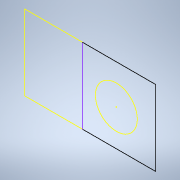
# Autodesk Inventor part: Palanca servo_dedo_2
Saved by Autodesk Inventor 2020 (Build 240168000, 168)
## iProperties
Created: 2021-08-17
Part Number: Palanca servo_dedo_2
Material: Generic
Document SubType Name: Modeling
Designer: chalo
Density: 1 g/cm^3
Appearance: Default
Author: chalo
Autodesk Inventor part; units mm, degrees
ref_plane "YZ Plane" through (0, 0, 0) normal (1, 0, 0) x (0, 1, 0)
ref_plane "XZ Plane" through (0, 0, 0) normal (0, 1, 0) x (-1, 0, 0)
ref_plane "XY Plane" through (0, 0, 0) normal (0, 0, 1) x (1, 0, 0)
sketch "Sketch1" plane through (0, 0, 0) normal (0, 0, 1) x (1, 0, 0)
  circle A0 centre (-2.5, -3) radius 1.6 projected
  line L0 (-10, -5.75) -> (0, -5.75) projected
  line L1 (0, 0) -> (0, -5.75) projected
  line L2 (-10, 0) -> (0, 0) projected
  line L3 (-10, -2) -> (-10, 0) projected
  line L4 (-10, -2) -> (-10, -3.75) projected
  line L5 (-10, -5.75) -> (-10, -3.75) projected
  line L6 (0, -5.75) -> (-5, -5.75)
  line L7 (-5, -5.75) -> (-5, 0)
  line L8 (-5, 0) -> (0, 0)
  line L9 (0, 0) -> (0, -5.75)
  dimension "d0" = 2.5
  constraints: 8 end point, 2 parallel, 1 horizontal, 1 midpoint, 1 perpendicular
  measures "d0" distance from line of A0.centre L7
extrude "Extrusion1" add sketch "Sketch1" along normal blind 4 contours L7 L2 L1 L0
sketch "Sketch2" plane through (-5, 0, 0) normal (0, 1, 0) x (1, 0, 0)
  line L0 (5, 0) -> (0, 0) projected
  line L1 (0, 0) -> (0, -4) projected
  line L2 (5, -4) -> (0, -4) projected
  line L3 (5, 0) -> (5, -4) projected
  line L4 (24.0211, -5.907) -> (18.6171, -5.907) projected
  line L5 (24.0211, -17.407) -> (18.6171, -17.407) projected
  line L6 (5, -4) -> (18.0171, -13.657)
  line L7 (5, 0) -> (18.0171, -9.657)
  line L8 (18.6171, -17.407) -> (18.6171, -13.657) construction
  line L9 (18.6171, -5.907) -> (18.6171, -9.657) construction
  line L10 (18.6171, -9.657) -> (18.6171, -13.657) construction
  line L11 (24.0211, -5.907) -> (24.0211, -17.407) construction
  line L12 (18.0171, -9.657) -> (26.5171, -9.657)
  line L13 (18.0171, -13.657) -> (26.5171, -13.657)
  line L14 (26.5171, -13.657) -> (26.5171, -9.657)
  line L15 (20.0171, -11.057) -> (20.0171, -5.657) construction
  point P0 (24.0211, -11.657)
  point P1 (18.6171, -11.657)
  dimension "d3" = 4
  dimension "d4" = 8.5
  dimension "d7" = 2
  constraints: 18 end point, 4 vertical, 3 horizontal alignment, 3 perpendicular, 2 midpoint, 1 vertical alignment
  measures "d3" distance of L9.end L8.end
  measures "d4" distance of L7.end L12.end
  measures "d7" distance from line of L15 L7.end
extrude "Extrusion2" add sketch "Sketch2" against normal blind 10 contours L7 L12 L14 L13 L6 L3
sketch "Sketch3" plane through (13.0171, 0, 13.657) normal (0, 0, 1) x (1, 0, 0)
  circle A0 centre (4.6, -6.8) radius 1.55 construction
  line L0 (-13.0171, 0) -> (0, 0) construction
  line L1 (-13.0171, -5.75) -> (-13.0171, 0) projected
  line L2 (-13.0171, -5.75) -> (-13.0171, -10) projected
  line L3 (0, -10) -> (-13.0171, -10) projected
  line L4 (0, 0) -> (0, -10) construction
  line L5 (0, 0) -> (8.5, 0) projected
  line L6 (0, 0) -> (0, -10) construction
  line L7 (8.5, -10) -> (0, -10) construction
  line L8 (8.5, 0) -> (8.5, -10) projected
  line L9 (-18.0171, -5.75) -> (-13.0171, -5.75) projected
  line L10 (-13.0171, -5.75) -> (-9.0171, -5.75)
  line L11 (-9.0171, -5.75) -> (1.6, -10)
  line L12 (8.5, -10) -> (0, -10) projected
  line L13 (-13.0171, 0) -> (-18.0171, 0) projected
  line L14 (-13.0171, 0) -> (-9.0171, 0)
  line L15 (0, 0) -> (-13.0171, 0) projected
  line L16 (-9.0171, 0) -> (1.6, -4.25)
  line L17 (1.6, -4.25) -> (7.6, -4.25)
  line L18 (7.6, -4.25) -> (7.6, -10)
  line L19 (2.7105, -10) -> (7.6, -10)
  dimension "d8" = 4
  dimension "d9" = 4
  dimension "d11" = 3
  dimension "d12" = 3
  constraints: 14 end point, 3 point on line, 2 horizontal, 1 collinear, 1 parallel, 1 perpendicular, 1 vertical alignment
  measures "d8" distance of L1.start L10.end
  measures "d9" distance of L13.start L14.end
  measures "d11" distance from line of L18 A0.centre
  measures "d12" horizontal distance of L16.end A0.centre
extrude "Extrusion3" cut sketch "Sketch3" against normal through all contours L10 L11 L12 L3 L2 | L15 L5 L8 L12 L18 L17 L16
sketch "Sketch4" plane through (14.6171, -10, 13.657) normal (0, 0, 1) x (1, 0, 0)
  line L0 (-1.6, 0.6405) -> (0, 0) projected
  line L1 (6, 0) -> (0, 0) projected
  line L2 (6, 0) -> (6, 5.75) projected
  line L3 (6, 5.75) -> (0, 5.75) projected
  line L4 (0, 5.75) -> (-1.6, 6.3905) projected
  line L5 (-1.6, 6.3905) -> (-1.6, 0.6405) projected
  circle A0 centre (3, 3.2) radius 1.55 projected
  point P0 (-14.6171, 10)
extrude "Extrusion4" cut sketch "Sketch4" against normal through all contours A0
body "Solid1"
